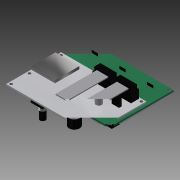
# Autodesk Inventor part: GLCDKnockoff
Saved by Autodesk Inventor 2015 SP1 (Build 190203100, 203)
## iProperties
Created: 2015-04-16
Part Number: GLCDKnockoff
Material: Generic
Document SubType Name: Modeling
Designer: Jack
Density: 1 g/cm^3
Appearance: Default
Author: Jack
Autodesk Inventor part; units mm, degrees
ref_plane "YZ Plane" through (0, 0, 0) normal (1, 0, 0) x (0, 1, 0)
ref_plane "XZ Plane" through (0, 0, 0) normal (0, 1, 0) x (-1, 0, 0)
ref_plane "XY Plane" through (0, 0, 0) normal (0, 0, 1) x (1, 0, 0)
sketch "Sketch1" plane through (0, 0, 0) normal (0, 0, 1) x (1, 0, 0)
  line L0 (0, 0) -> (93, 0)
  line L1 (93, 0) -> (93, 60)
  line L2 (93, 60) -> (0, 60)
  line L3 (0, 60) -> (0, 0)
  dimension "d0" = 93
  dimension "d1" = 60
  constraints: 8 end point, 2 parallel, 1 horizontal, 1 perpendicular
  measures "d0" distance of L2.end L1.end
  measures "d1" distance of L1.end L0.end
extrude "ControlPCB" add sketch "Sketch1" along normal blind 1.65
ref_plane "Work Plane1" through (0, 0, -2.6) normal (0, 0, -1) x (-1, 0, 0)
sketch "Sketch2" plane through (0, 0, -2.6) normal (0, 0, -1) x (-1, 0, 0)
  line L0 (-93, 0) -> (-93, 60) projected
  line L1 (-93, 20) -> (0, 20)
  line L2 (0, 20) -> (0, 90)
  line L3 (0, 90) -> (-93, 90)
  line L4 (-93, 90) -> (-93, 20)
  line L5 (0, 0) -> (-93, 0) projected
  dimension "d5" = 70
  dimension "d6" = 20
  constraints: 8 end point, 2 parallel, 1 horizontal, 1 perpendicular, 1 point on line, 1 vertical alignment
  measures "d5" distance of L1.end L2.end
  measures "d6" distance between parallel lines of L5 L1
extrude "LCDPCB" add sketch "Sketch2" along normal blind 1.65
sketch "Sketch3" plane through (0, 0, 0) normal (0, 0, -1) x (-1, 0, 0)
  line L0 (0, 0) -> (-93, 0) projected
  line L1 (0, 60) -> (0, 0) projected
  line L2 (-93, 60) -> (0, 60) projected
  line L3 (-93, 0) -> (-93, 60) projected
  point P0 (-90.25, 2.75)
  point P1 (-2.75, 2.75)
  point P2 (-90.25, 22.75)
  point P3 (-2.75, 22.75)
  point P4 (-90.25, 57.25)
  point P5 (-2.75, 57.25)
  dimension "d9" = 2.75
  dimension "d10" = 2.75
  dimension "d11" = 2.75
  dimension "d12" = 2.75
  dimension "d13" = 22.75
  constraints: 4 vertical alignment, 3 horizontal alignment
  measures "d9" distance from line of L3 point (-90.25, 2.75)
  measures "d10" distance from line of point (-90.25, 2.75) L0
  measures "d11" distance from line of L2 point (-90.25, 57.25)
  measures "d12" distance from line of L1 point (-2.75, 57.25)
  measures "d13" distance from line of L0 point (-2.75, 22.75)
hole "ControlPCBHoles" at (90.25, 2.75, 0) at (2.75, 2.75, 0) at (90.25, 22.75, 0) at (2.75, 22.75, 0) at (90.25, 57.25, 0) at (2.75, 57.25, 0) direction (0, 0, 1) diameter 3 end up to face face through (62, 20, 1.65) facing (0, 0, 1)
sketch "Sketch4" plane through (0, 0, -4.25) normal (0, 0, -1) x (-1, 0, 0)
  line L0 (0, 90) -> (-93, 90) projected
  circle A0 centre (-90.25, 22.75) radius 1.5 projected
  circle A1 centre (-2.75, 22.75) radius 1.5 projected
  point P0 (0, 0)
  point P1 (-90.25, 87.25)
  point P2 (-2.75, 87.25)
  dimension "d21" = 2.75
  constraints: 2 vertical alignment, 1 horizontal alignment
  measures "d21" distance from line of L0 point (-90.25, 87.25)
hole "LCDPCBHoles" at (90.25, 87.25, -4.25) at (2.75, 87.25, -4.25) at (90.25, 22.75, -4.25) at (2.75, 22.75, -4.25) direction (0, 0, 1) diameter 3 end up to face face through (62, 43.3333, -2.6) facing (0, 0, 1)
sketch "Sketch5" plane through (0, 0, 0) normal (0, 0, -1) x (-1, 0, 0)
  line L0 (0, 0) -> (-93, 0) projected
  line L1 (0, 60) -> (0, 0) projected
  line L2 (-14.7, 5) -> (-8.7, 5)
  line L3 (-8.7, 5) -> (-8.7, 11)
  line L4 (-8.7, 11) -> (-14.7, 11)
  line L5 (-14.7, 11) -> (-14.7, 5)
  line L6 (-46.8, 5) -> (-40.8, 5)
  line L7 (-40.8, 5) -> (-40.8, 11)
  line L8 (-40.8, 11) -> (-46.8, 11)
  line L9 (-46.8, 11) -> (-46.8, 5)
  dimension "d29" = 6
  dimension "d30" = 6
  dimension "d31" = 6
  dimension "d32" = 6
  dimension "d33" = 5
  dimension "d34" = 8.7
  dimension "d35" = 46.8
  constraints: 16 end point, 4 parallel, 2 horizontal, 2 perpendicular, 1 horizontal alignment
  measures "d29" distance of L4.end L3.end
  measures "d30" distance of L3.end L2.end
  measures "d31" distance of L8.end L7.end
  measures "d32" distance of L7.end L6.end
  measures "d33" distance between parallel lines of L0 L2
  measures "d34" distance between parallel lines of L1 L3
  measures "d35" distance between parallel lines of L1 L9
extrude "FrontButtonBody" add sketch "Sketch5" along normal blind 4
sketch "Sketch6" plane through (0, 0, -4) normal (0, 0, -1) x (-1, 0, 0)
  line L0 (-8.7, 5) -> (-8.7, 11) projected
  line L1 (-8.7, 11) -> (-14.7, 11) projected
  line L2 (-46.8, 5) -> (-40.8, 5) projected
  line L3 (-40.8, 5) -> (-40.8, 11) projected
  line L4 (-40.8, 11) -> (-46.8, 11) projected
  line L5 (-46.8, 11) -> (-46.8, 5) projected
  circle A0 centre (-43.8, 8) radius 1.75
  circle A1 centre (-11.7, 8) radius 1.75
  point P0 (0, 0)
  dimension "d38" = 3.5
  dimension "d39" = 3
  dimension "d40" = 3
  dimension "d41" = 3
  dimension "d42" = 3
  constraints: 2 centre point, 1 equal radius
  measures "d38" diameter of A0
  measures "d39" distance from line of L1 A1.centre
  measures "d40" distance from line of L0 A1.centre
  measures "d41" distance from line of L3 A0.centre
  measures "d42" distance from line of L2 A0.centre
extrude "FrontButtonTop" add sketch "Sketch6" along normal blind 1.6 contours A0 | A1
sketch "Sketch7" plane through (0, 0, 0) normal (0, 0, -1) x (-1, 0, 0)
  line L0 (0, 0) -> (-93, 0) projected
  line L1 (-93, 0) -> (-93, 60) projected
  circle A0 centre (-65, 9.4) radius 5.8
  dimension "d45" = 11.6
  dimension "d46" = 28
  dimension "d47" = 9.4
  constraints: 1 centre point
  measures "d45" diameter of A0
  measures "d46" distance from line of L1 A0.centre
  measures "d47" distance from line of L0 A0.centre
extrude "Buzzer" add sketch "Sketch7" along normal blind 9.6
sketch "Sketch8" plane through (0, 0, 0) normal (0, 0, -1) x (-1, 0, 0)
  line L0 (0, 0) -> (-93, 0) projected
  line L1 (0, 60) -> (0, 0) projected
  line L2 (-15.5, 13.6) -> (-10.5, 13.6)
  line L3 (-10.5, 13.6) -> (-10.5, 18.6)
  line L4 (-10.5, 18.6) -> (-15.5, 18.6)
  line L5 (-15.5, 18.6) -> (-15.5, 13.6)
  dimension "d50" = 5
  dimension "d51" = 5
  dimension "d52" = 13.6
  dimension "d53" = 10.5
  constraints: 8 end point, 2 parallel, 1 horizontal, 1 perpendicular
  measures "d50" distance of L4.end L3.end
  measures "d51" distance of L3.end L2.end
  measures "d52" distance between parallel lines of L0 L2
  measures "d53" distance between parallel lines of L1 L3
extrude "FrontPot" add sketch "Sketch8" along normal blind 2
sketch "Sketch9" plane through (0, 0, -2) normal (0, 0, -1) x (-1, 0, 0)
  line L0 (-15.5, 13.6) -> (-10.5, 13.6) projected
  line L1 (-10.5, 13.6) -> (-10.5, 18.6) projected
  line L2 (-13.4, 15.7) -> (-13.4, 14.95)
  line L3 (-13.4, 14.95) -> (-12.6, 14.95)
  line L4 (-12.6, 14.95) -> (-12.6, 15.7)
  line L5 (-12.6, 15.7) -> (-11.85, 15.7)
  line L6 (-11.85, 15.7) -> (-11.85, 16.5)
  line L7 (-11.85, 16.5) -> (-12.6, 16.5)
  line L8 (-12.6, 16.5) -> (-12.6, 17.25)
  line L9 (-12.6, 17.25) -> (-13.4, 17.25)
  line L10 (-13.4, 17.25) -> (-13.4, 16.5)
  line L11 (-14.15, 16.5) -> (-14.15, 15.7)
  line L12 (-14.15, 15.7) -> (-13.4, 15.7)
  line L13 (-13.4, 16.5) -> (-14.15, 16.5)
  point P0 (0, 0)
  dimension "d56" = 0.8
  dimension "d57" = 2.3
  dimension "d58" = 2.1
  dimension "d59" = 2.1
  constraints: 24 end point, 7 perpendicular, 7 point on line, 4 equal length, 2 parallel, 1 vertical
  measures "d56" distance between parallel lines of L5 L7
  measures "d57" distance between parallel lines of L11 L6
  measures "d58" distance between parallel lines of L1 L8
  measures "d59" distance between parallel lines of L0 L5
extrude "FrontPotScrewHole" cut sketch "Sketch9" against normal blind 0.8
sketch "Sketch10" plane through (0, 0, 0) normal (0, 0, -1) x (-1, 0, 0)
  line L0 (0, 0) -> (-93, 0) projected
  line L1 (0, 60) -> (0, 0) projected
  line L2 (-35.9, 3.7) -> (-23.2, 3.7)
  line L3 (-23.2, 3.7) -> (-23.2, 17.1)
  line L4 (-23.2, 17.1) -> (-35.9, 17.1)
  line L5 (-35.9, 17.1) -> (-35.9, 3.7)
  dimension "d62" = 12.7
  dimension "d63" = 13.4
  dimension "d64" = 3.7
  dimension "d65" = 23.2
  constraints: 8 end point, 2 parallel, 1 horizontal, 1 perpendicular
  measures "d62" distance of L4.end L3.end
  measures "d63" distance of L3.end L2.end
  measures "d64" distance between parallel lines of L0 L2
  measures "d65" distance between parallel lines of L3 L1
extrude "EncoderBase" add sketch "Sketch10" along normal blind 6.2
sketch "Sketch11" plane through (0, 0, -6.2) normal (0, 0, -1) x (-1, 0, 0)
  line L0 (-23.2, 17.1) -> (-35.9, 17.1) projected
  line L1 (-35.9, 17.1) -> (-35.9, 3.7) projected
  circle A0 centre (-29.55, 10.4) radius 3.4
  point P0 (0, 0)
  dimension "d68" = 6.8
  dimension "d69" = 6.7
  dimension "d70" = 6.35
  constraints: 1 centre point
  measures "d68" diameter of A0
  measures "d69" distance from line of L0 A0.centre
  measures "d70" distance from line of L1 A0.centre
extrude "EncoderShaftSupport" add sketch "Sketch11" along normal blind 6.4
sketch "Sketch12" plane through (29.55, 10.4, -12.6) normal (0, 0, -1) x (-1, 0, 0)
  circle A0 centre (0, 0) radius 3.4 projected
  circle A1 centre (0, 0) radius 3
  line L0 (0, 3) -> (2.5981, -1.5)
  line L1 (0, 0) -> (0, -3) construction
  point P0 (29.55, -10.4)
  dimension "d73" = 6
  dimension "d74" = 1.5
  dimension "d75" = 30
  constraints: 4 end point, 3 point on circle, 1 centre point, 1 coincident, 1 vertical
  measures "d73" diameter of A1
  measures "d74" distance from line of A0.centre L0
  measures "d75" angle of L0 L1
extrude "EncoderShaft" add sketch "Sketch12" along normal blind 9.2 contours L0 A1 picked at (-0.0801, -0.2988)
sketch "Sketch13" plane through (0, 0, -4.25) normal (0, 0, -1) x (-1, 0, 0)
  line L0 (-93, 20) -> (0, 20) projected
  line L1 (0, 20) -> (0, 90) projected
  line L2 (-81, 20.5) -> (-30, 20.5)
  line L3 (-30, 20.5) -> (-30, 24.5)
  line L4 (-30, 24.5) -> (-81, 24.5)
  line L5 (-81, 24.5) -> (-81, 20.5)
  point P0 (0, 0)
  dimension "d78" = 4
  dimension "d79" = 51
  dimension "d80" = 30
  dimension "d81" = 0.5
  constraints: 8 end point, 2 parallel, 1 horizontal, 1 perpendicular
  measures "d78" distance of L2.end L3.end
  measures "d79" distance of L2.start L2.end
  measures "d80" distance between parallel lines of L1 L3
  measures "d81" distance between parallel lines of L0 L2
extrude "LCDPins" add sketch "Sketch13" along normal blind 1.7
sketch "Sketch14" plane through (0, 0, -4.25) normal (0, 0, -1) x (-1, 0, 0)
  line L0 (0, 20) -> (0, 90) projected
  line L1 (0, 90) -> (-93, 90) projected
  line L2 (-85.7, 29.6) -> (-7.7, 29.6)
  line L3 (-7.7, 29.6) -> (-7.7, 80.6)
  line L4 (-7.7, 80.6) -> (-85.7, 80.6)
  line L5 (-85.7, 80.6) -> (-85.7, 29.6)
  point P0 (0, 0)
  dimension "d84" = 78
  dimension "d85" = 51
  dimension "d86" = 7.7
  dimension "d87" = 9.4
  constraints: 8 end point, 2 parallel, 1 horizontal, 1 perpendicular
  measures "d84" distance of L4.end L3.end
  measures "d85" distance of L3.end L2.end
  measures "d86" distance between parallel lines of L0 L3
  measures "d87" distance between parallel lines of L1 L4
extrude "LCD" add sketch "Sketch14" along normal blind 8.5
sketch "Sketch15" plane through (0, 0, -12.75) normal (0, 0, -1) x (-1, 0, 0)
  line L0 (-85.7, 29.6) -> (-7.7, 29.6) projected
  line L1 (-85.7, 80.6) -> (-85.7, 29.6) projected
  line L2 (-82.7, 35.1) -> (-10.7, 35.1)
  line L3 (-10.7, 35.1) -> (-10.7, 75.1)
  line L4 (-10.7, 75.1) -> (-82.7, 75.1)
  line L5 (-82.7, 75.1) -> (-82.7, 35.1)
  point P0 (0, 0)
  dimension "d90" = 72
  dimension "d91" = 40
  dimension "d92" = 5.5
  dimension "d93" = 3
  constraints: 8 end point, 2 parallel, 1 horizontal, 1 perpendicular
  measures "d90" distance of L4.end L3.end
  measures "d91" distance of L3.end L2.end
  measures "d92" distance between parallel lines of L0 L2
  measures "d93" distance between parallel lines of L1 L5
extrude "LCDIndent" cut sketch "Sketch15" against normal blind 1
sketch "Sketch16" plane through (0, 0, -4.25) normal (0, 0, -1) x (-1, 0, 0)
  line L0 (-85.7, 29.6) -> (-85.7, 80.6) projected
  line L1 (-7.7, 29.6) -> (-85.7, 29.6) projected
  line L2 (-85.7, 33.6) -> (-91.1, 33.6)
  line L3 (-91.1, 33.6) -> (-91.1, 76.6)
  line L4 (-91.1, 76.6) -> (-85.7, 76.6)
  line L5 (-85.7, 76.6) -> (-85.7, 33.6)
  point P0 (0, 0)
  dimension "d96" = 5.4
  dimension "d97" = 43
  dimension "d98" = 4
  constraints: 8 end point, 2 parallel, 1 horizontal, 1 perpendicular, 1 point on line
  measures "d96" distance of L3.end L4.end
  measures "d97" distance of L2.end L3.end
  measures "d98" distance between parallel lines of L1 L2
extrude "BackLight" add sketch "Sketch16" along normal blind 3.4
sketch "Sketch17" plane through (0, 0, -2.6) normal (0, 0, 1) x (1, 0, 0)
  line L0 (93, 90) -> (93, 20) projected
  line L1 (0, 90) -> (93, 90) projected
  line L2 (0, 20) -> (0, 90) projected
  line L3 (13, 80.3) -> (19.5, 80.3)
  line L4 (19.5, 80.3) -> (19.5, 80.8)
  line L5 (19.5, 80.8) -> (13, 80.8)
  line L6 (13, 80.8) -> (13, 80.3)
  line L7 (73.5, 80.3) -> (80, 80.3)
  line L8 (80, 80.3) -> (80, 80.8)
  line L9 (80, 80.8) -> (73.5, 80.8)
  line L10 (73.5, 80.8) -> (73.5, 80.3)
  line L11 (43.25, 80.3) -> (49.75, 80.3)
  line L12 (49.75, 80.3) -> (49.75, 80.8)
  line L13 (49.75, 80.8) -> (43.25, 80.8)
  line L14 (43.25, 80.8) -> (43.25, 80.3)
  point P0 (0, 0)
  dimension "d101" = 6.5
  dimension "d102" = 0.5
  dimension "d103" = 6.5
  dimension "d104" = 0.5
  dimension "d105" = 6.5
  dimension "d106" = 0.5
  dimension "d107" = 13
  dimension "d108" = 13
  dimension "d109" = 43.25
  dimension "d110" = 9.2
  constraints: 24 end point, 6 parallel, 3 horizontal, 3 perpendicular, 2 horizontal alignment
  measures "d101" distance of L5.end L4.end
  measures "d102" distance of L4.end L3.end
  measures "d103" distance of L9.end L8.end
  measures "d104" distance of L8.end L7.end
  measures "d105" distance of L13.end L12.end
  measures "d106" distance of L12.end L11.end
  measures "d107" distance between parallel lines of L2 L6
  measures "d108" distance between parallel lines of L0 L8
  measures "d109" distance between parallel lines of L0 L12
  measures "d110" distance between parallel lines of L13 L1
extrude "LCDTabs" add sketch "Sketch17" along normal blind 2.5
sketch "Sketch18" plane through (0, 0, 1.65) normal (0, 0, 1) x (1, 0, 0)
  line L0 (93, 60) -> (0, 60) projected
  line L1 (0, 60) -> (0, 0) projected
  line L2 (0, 27.3) -> (26, 27.3)
  line L3 (26, 27.3) -> (26, 53.8)
  line L4 (26, 53.8) -> (0, 53.8)
  line L5 (0, 53.8) -> (0, 27.3)
  dimension "d113" = 26
  dimension "d114" = 26.5
  dimension "d115" = 6.2
  constraints: 8 end point, 2 parallel, 1 collinear, 1 horizontal, 1 perpendicular
  measures "d113" distance of L4.end L3.end
  measures "d114" distance of L3.end L2.end
  measures "d115" distance between parallel lines of L0 L4
extrude "SDSlotBody" add sketch "Sketch18" along normal blind 3
sketch "Sketch20" plane through (0, 0, 1.65) normal (0, 0, 1) x (1, 0, 0)
  line L0 (93, 0) -> (93, 60) projected
  line L1 (93, 60) -> (0, 60) projected
  line L2 (44, 49.9) -> (64.4, 49.9)
  line L3 (64.4, 49.9) -> (64.4, 58.7)
  line L4 (64.4, 58.7) -> (44, 58.7)
  line L5 (44, 58.7) -> (44, 49.9)
  line L6 (66, 58.7) -> (86.4, 58.7)
  line L7 (86.4, 58.7) -> (86.4, 49.9)
  line L8 (86.4, 49.9) -> (66, 49.9)
  line L9 (66, 49.9) -> (66, 58.7)
  dimension "d124" = 20.4
  dimension "d125" = 8.8
  dimension "d126" = 6.6
  dimension "d127" = 1.3
  dimension "d128" = 1.6
  constraints: 16 end point, 4 parallel, 2 horizontal, 2 perpendicular, 2 point on line, 1 collinear, 1 horizontal alignment
  measures "d124" distance of L6.start L6.end
  measures "d125" distance of L6.end L7.end
  measures "d126" distance between parallel lines of L0 L7
  measures "d127" distance between parallel lines of L1 L6
  measures "d128" distance between parallel lines of L9 L3
extrude "IOConnectors" add sketch "Sketch20" along normal blind 9
sketch "Sketch21" plane through (0, 0, 1.65) normal (0, 0, 1) x (1, 0, 0)
  line L0 (93, 0) -> (93, 60) projected
  line L1 (93, 60) -> (0, 60) projected
  line L2 (76.2, 39) -> (84.2, 39)
  line L3 (84.2, 39) -> (84.2, 42)
  line L4 (84.2, 42) -> (76.2, 42)
  line L5 (76.2, 42) -> (76.2, 39)
  dimension "d131" = 8
  dimension "d132" = 3
  dimension "d133" = 8.8
  dimension "d134" = 18
  constraints: 8 end point, 2 parallel, 1 horizontal, 1 perpendicular
  measures "d131" distance of L4.end L3.end
  measures "d132" distance of L3.end L2.end
  measures "d133" distance between parallel lines of L0 L3
  measures "d134" distance between parallel lines of L1 L4
extrude "MiscHeader" add sketch "Sketch21" along normal blind 8.5
sketch "Sketch22" plane through (0, 0, 1.65) normal (0, 0, 1) x (1, 0, 0)
  line L0 (0, 0) -> (93, 0) projected
  line L1 (93, 0) -> (93, 60) projected
  circle A0 centre (68.8, 32.4) radius 3.2
  dimension "d137" = 6.4
  dimension "d138" = 24.2
  dimension "d139" = 32.4
  constraints: 1 centre point
  measures "d137" diameter of A0
  measures "d138" distance from line of L1 A0.centre
  measures "d139" distance from line of A0.centre L0
extrude "RearCap" add sketch "Sketch22" along normal blind 8
sketch "Sketch23" plane through (0, 0, 10.65) normal (0, 0, 1) x (1, 0, 0)
  line L0 (44, 49.9) -> (64.4, 49.9) projected
  line L1 (64.4, 49.9) -> (64.4, 58.7) projected
  line L2 (64.4, 58.7) -> (44, 58.7) projected
  line L3 (44, 58.7) -> (44, 49.9) projected
  line L4 (86.4, 58.7) -> (66, 58.7) projected
  line L5 (66, 58.7) -> (66, 49.9) projected
  line L6 (66, 49.9) -> (86.4, 49.9) projected
  line L7 (86.4, 49.9) -> (86.4, 58.7) projected
  line L8 (45.2, 57.5) -> (63.2, 57.5)
  line L9 (63.2, 57.5) -> (63.2, 51.1)
  line L10 (63.2, 51.1) -> (45.2, 51.1)
  line L11 (45.2, 51.1) -> (45.2, 57.5)
  line L12 (67.2, 57.5) -> (85.2, 57.5)
  line L13 (85.2, 57.5) -> (85.2, 51.1)
  line L14 (85.2, 51.1) -> (67.2, 51.1)
  line L15 (67.2, 51.1) -> (67.2, 57.5)
  point P0 (0, 0)
  dimension "d146" = 1.2
  dimension "d147" = 1.2
  constraints: 16 end point, 6 other
  measures "d146" distance between parallel lines of L4 L12
  measures "d147" distance between parallel lines of L1 L9
extrude "CableEnd" add sketch "Sketch23" along normal blind 4.6 contours L8 L9 L10 L11 | L12 L13 L14 L15
sketch "Sketch24" plane through (45.2, 51.1, 10.65) normal (0, -1, 0) x (1, 0, 0)
  line L0 (0, 4.6) -> (18, 4.6) projected
  line L1 (0, 0) -> (0, 4.6) projected
  line L2 (40, 0) -> (22, 0) projected
  line L3 (40, 0) -> (40, 4.6) projected
  line L4 (22, 4.6) -> (40, 4.6) projected
  line L5 (22, 0) -> (22, 4.6) projected
  line L6 (2.65, 1.6) -> (15.35, 1.6)
  line L7 (15.35, 1.6) -> (15.35, 2.6)
  line L8 (15.35, 2.6) -> (2.65, 2.6)
  line L9 (2.65, 2.6) -> (2.65, 1.6)
  line L10 (24.65, 1.6) -> (37.35, 1.6)
  line L11 (37.35, 1.6) -> (37.35, 2.6)
  line L12 (37.35, 2.6) -> (24.65, 2.6)
  line L13 (24.65, 2.6) -> (24.65, 1.6)
  point P0 (-45.2, -10.65)
  dimension "d150" = 2
  dimension "d151" = 1
  dimension "d152" = 12.7
  dimension "d153" = 2.65
  dimension "d154" = 2.65
  constraints: 16 end point, 4 parallel, 2 equal length, 2 horizontal, 2 perpendicular, 1 horizontal alignment
  measures "d150" distance between parallel lines of L0 L8
  measures "d151" distance of L6.end L7.end
  measures "d152" distance of L7.end L8.end
  measures "d153" distance between parallel lines of L1 L9
  measures "d154" distance between parallel lines of L5 L13
extrude "Cable" add sketch "Sketch24" along normal blind 45 contours L9 L8 L7 L6 | L13 L12 L11 L10
body "Solid1"
